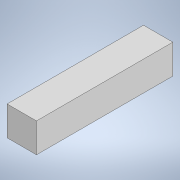
# Autodesk Inventor part: rail part
Saved by Autodesk Inventor 2021 (Build 250183000, 183)
## iProperties
Created: 2021-04-19
Part Number: rail part
Material: Generic
Document SubType Name: Modeling
Designer: miw14
Density: 1 g/cm^3
Appearance: Default
Author: miw14
Autodesk Inventor part; units mm, degrees
ref_plane "YZ Plane" through (0, 0, 0) normal (1, 0, 0) x (0, 1, 0)
ref_plane "XZ Plane" through (0, 0, 0) normal (0, 1, 0) x (-1, 0, 0)
ref_plane "XY Plane" through (0, 0, 0) normal (0, 0, 1) x (1, 0, 0)
sketch "Sketch1" plane through (0, 0, 0) normal (0, 0, 1) x (1, 0, 0)
  line L0 (165.1, 0) -> (165.1, 165.1)
  line L1 (165.1, 165.1) -> (0, 165.1)
  line L2 (0, 165.1) -> (0, 0)
  line L3 (-15.875, -15.875) -> (180.975, -15.875)
  line L4 (180.975, -15.875) -> (180.975, 180.975)
  line L5 (180.975, 180.975) -> (-15.875, 180.975)
  line L6 (-15.875, 180.975) -> (-15.875, -15.875)
  line L7 (-15.875, -15.875) -> (180.975, -15.875)
  line L8 (180.975, -15.875) -> (180.975, 3.178)
  line L9 (180.975, 3.178) -> (-15.875, 3.178)
  line L10 (-15.875, 3.178) -> (-15.875, -15.875)
  dimension "d7" = 196.85
  dimension "d8" = 196.85
  dimension "d9" = 15.875
  dimension "d10" = 196.85
  dimension "d11" = 15.875
  constraints: 22 end point, 5 parallel, 2 horizontal, 2 perpendicular
  measures "d7" distance of L4.end L5.end
  measures "d8" distance of L8.end L9.end
  measures "d9" distance between parallel lines of L4 L0
  measures "d10" distance of L3.end L4.end
  measures "d11" distance between parallel lines of L1 L5
extrude "Extrusion1" add sketch "Sketch1" along normal blind 914.4
body "Solid1"
